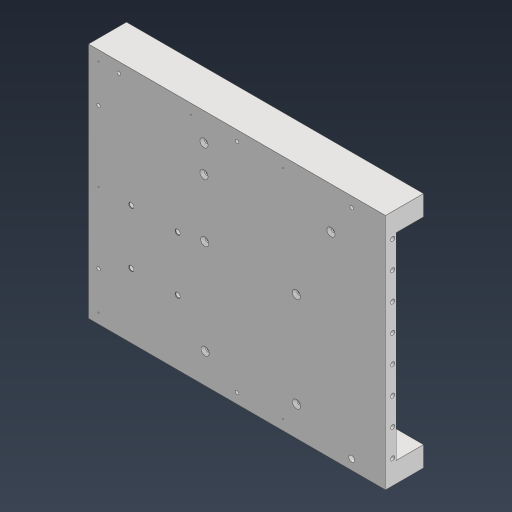
# Autodesk Inventor part: case1
Saved by Autodesk Inventor 2023 (Build 270158000, 158)
## iProperties
Created: 2026-01-23
Part Number: case1
Material: Generic
Document SubType Name: Modeling
Designer: szymo
Density: 1 g/cm^3
Appearance: Default
Author: szymo
Autodesk Inventor part; units mm, degrees
sketch "Sketch1" plane through (0, 0, 0) normal (0, 0, 1) x (1, 0, 0)
  line L0 (100, -105) -> (100, 95)
  line L1 (100, 95) -> (-150, 95)
  line L2 (-150, 95) -> (-150, -105)
  line L3 (-150, -105) -> (100, -105)
  line L4 (-150, -105) -> (-400, -105)
  line L5 (-400, -105) -> (-400, 95)
  line L6 (-400, 95) -> (-150, 95)
  line L7 (-150, 95) -> (-150, -105)
  line L8 (-150, -88) -> (-400, -88)
  line L9 (-400, 78) -> (-150, 78)
  line L10 (-150, -88) -> (83, -88)
  line L11 (83, 78) -> (-150, 78)
  line L12 (-150, 78) -> (-150, 78)
  line L13 (-150, -88) -> (-150, -88)
  line L14 (-383, -105) -> (-383, 95)
  circle A0 centre (13.833333, -96.5) radius 0.5
  circle A1 centre (91.5, 86.5) radius 0.5
  circle A2 centre (91.5, -96.5) radius 0.5
  circle A3 centre (-63.833333, -96.5) radius 0.5
  circle A4 centre (91.5, -5) radius 0.5
  circle A5 centre (13.833333, 86.5) radius 0.5
  circle A6 centre (-63.833333, 86.5) radius 0.5
  circle A7 centre (-121.5, 86.5) radius 1.5
  circle A8 centre (-25, -96.5) radius 1.5
  circle A9 centre (91.5, 40.75) radius 1.5
  circle A10 centre (74.5, -96.5) radius 1.5
  circle A11 centre (91.5, -50.75) radius 1.5
  circle A12 centre (74.5, 86.5) radius 1.5
  circle A13 centre (-121.5, -96.5) radius 1.5
  circle A14 centre (-25, 86.5) radius 1.5
  point P0 (0, 0)
  point P1 (-125, 125)
  point P2 (-127, 93)
  point P3 (-127, 93)
  point P4 (105, -105)
  point P5 (-383, -88)
  point P6 (-383, 78)
  dimension "d0" = 250
  dimension "d23" = 17
  dimension "d24" = 17
  constraints: 18 end point, 6 point on line, 4 perpendicular, 3 horizontal, 2 parallel
  measures "d0" distance of L1.end L5.end
  measures "d23" distance between parallel lines of L11 L1
  measures "d24" distance between parallel lines of L5 L14
ref_plane "Work Plane1" through (-125, -125, -32) normal (0, 0, -1) x (0, 1, 0)
ref_plane "Work Plane5" through (-127, -103, -32) normal (0, 0, -1) x (0, 1, 0)
extrude "Extrusion1" add sketch "Sketch1" against normal up to surface (32 mm away) contours L4 L14 L8 L2 | L2 L9 L14 L6 | L4 L5 L8 L14 | L14 L9 L5 L6 | L8 L5 L9 L14
ref_plane "Work Plane3" through (-122.5, -105, -3) normal (0, 0, -1) x (0, 1, 0)
sketch "Sketch2" plane through (0, 0, 0) normal (0, 0, 1) x (1, 0, 0)
  line L0 (100, 95) -> (100, -105)
  line L1 (100, -105) -> (-150, -105)
  line L2 (-150, -105) -> (-150, -88)
  line L3 (-150, -88) -> (83, -88)
  line L4 (83, -88) -> (83, 78)
  line L5 (83, 78) -> (-150, 78)
  line L6 (-150, 78) -> (-150, 95)
  line L7 (-150, 95) -> (100, 95)
  line L8 (-150, -105) -> (-400, -105)
  line L9 (-400, -105) -> (-400, 95)
  line L10 (-400, 95) -> (-150, 95)
  line L11 (-150, 95) -> (-150, -105)
  circle A0 centre (13.833333, -96.5) radius 0.5
  circle A1 centre (91.5, 86.5) radius 0.5
  circle A2 centre (91.5, -96.5) radius 0.5
  circle A3 centre (-63.833333, -96.5) radius 0.5
  circle A4 centre (91.5, -5) radius 0.5
  circle A5 centre (13.833333, 86.5) radius 0.5
  circle A6 centre (-63.833333, 86.5) radius 0.5
  circle A7 centre (-121.5, 86.5) radius 1.5
  circle A8 centre (-25, -96.5) radius 1.5
  circle A9 centre (91.5, 40.75) radius 1.5
  circle A10 centre (74.5, -96.5) radius 1.5
  circle A11 centre (91.5, -50.75) radius 1.5
  circle A12 centre (74.5, 86.5) radius 1.5
  circle A13 centre (-121.5, -96.5) radius 1.5
  circle A14 centre (-25, 86.5) radius 1.5
  point P0 (0, 0)
  dimension "d15" = 250
  constraints: 8 end point, 2 parallel, 1 horizontal, 1 perpendicular
  measures "d15" distance between parallel lines of L11 L9
extrude "Extrusion2" add sketch "Sketch2" against normal up to surface (3 mm away) contours L6 L11 L2 L8 L9 L10
sketch "Sketch6" plane through (-150, 78, -3) normal (0, 0, -1) x (-1, 0, 0)
  line L0 (0, 0) -> (233, 0) projected
  line L1 (0, -166) -> (0, 0) projected
  line L2 (233, -166) -> (0, -166) projected
  line L3 (0, -166) -> (233, -166) projected
  line L4 (0, -166) -> (2.5, -166)
  line L5 (2.5, -166) -> (2.5, 0)
  line L6 (2.5, 0) -> (0, 0)
  line L7 (0, 0) -> (0, -166)
  line L8 (36, -166) -> (66, -166)
  line L9 (66, 0) -> (36, 0)
  line L10 (17.5, -166) -> (32.5, -166)
  line L11 (32.5, -166) -> (32.5, 0)
  line L12 (32.5, 0) -> (17.5, 0)
  line L13 (17.5, 0) -> (17.5, -166)
  line L14 (233, 0) -> (233, -166) projected
  point P0 (-150, -78)
  point P1 (250, -164)
  point P2 (17.5, 0)
  point P3 (17.5, -166)
  point P4 (32.5, -166)
  point P5 (32.5, 0)
  dimension "d16" = 2.5
  dimension "d21" = 15
  dimension "d22" = 15
  constraints: 20 end point, 5 parallel, 3 horizontal, 3 point on line, 2 perpendicular, 3 other
  measures "d16" distance between parallel lines of L1 L5
  measures "d21" distance between parallel lines of L13 L5
  measures "d22" distance between parallel lines of L11 L13
ref_plane "Work Plane6" through (-94.5, -85, -9) normal (0, 0, -1) x (0, 1, 0)
extrude "Extrusion6" add sketch "Sketch6" along normal up to surface (6 mm away) contours L0 L5 L2 L1 | L0 L11 L2 L13
sketch "Sketch7" plane through (-400, -105, 0) normal (-1, 0, 0) x (0, 0, 1)
  line L0 (-32, 17) -> (-32, 183)
  line L1 (0, 0) -> (0, 200)
  line L2 (-32, 91.5) -> (0, 91.5)
  line L3 (0, 91.5) -> (0, 108.5)
  line L4 (0, 108.5) -> (-32, 108.5)
  line L5 (-32, 108.5) -> (-32, 91.5)
  line L6 (0, 0) -> (-32, 0)
  line L7 (0, 200) -> (-32, 200)
  line L8 (-22.75, 87.025535) -> (-15, 91.5)
  line L9 (-15, 91.5) -> (-7.25, 87.025535)
  line L10 (-7.25, 87.025535) -> (-7.25, 78.076606)
  line L11 (-7.25, 78.076606) -> (-15, 73.602142)
  line L12 (-15, 73.602142) -> (-22.75, 78.076606)
  line L13 (-22.75, 78.076606) -> (-22.75, 87.025535)
  line L14 (-22.75, 66.127677) -> (-15, 70.602142)
  line L15 (-15, 70.602142) -> (-7.25, 66.127677)
  line L16 (-7.25, 66.127677) -> (-7.25, 57.178748)
  line L17 (-7.25, 57.178748) -> (-15, 52.704283)
  line L18 (-15, 52.704283) -> (-22.75, 57.178748)
  line L19 (-22.75, 57.178748) -> (-22.75, 66.127677)
  line L20 (-22.75, 121.923394) -> (-15, 126.397858)
  line L21 (-15, 126.397858) -> (-7.25, 121.923394)
  line L22 (-7.25, 121.923394) -> (-7.25, 112.974465)
  line L23 (-7.25, 112.974465) -> (-15, 108.5)
  line L24 (-15, 108.5) -> (-22.75, 112.974465)
  line L25 (-22.75, 112.974465) -> (-22.75, 121.923394)
  line L26 (-22.75, 142.821252) -> (-15, 147.295717)
  line L27 (-15, 147.295717) -> (-7.25, 142.821252)
  line L28 (-7.25, 142.821252) -> (-7.25, 133.872323)
  line L29 (-7.25, 133.872323) -> (-15, 129.397858)
  line L30 (-15, 129.397858) -> (-22.75, 133.872323)
  line L31 (-22.75, 133.872323) -> (-22.75, 142.821252)
  line L32 (-3, 43.661423) -> (-3, 184.946283) construction
  point P0 (0, 105)
  point P1 (-15, 82.551071)
  point P2 (-15, 61.653212)
  point P3 (-15, 117.448929)
  point P4 (-15, 138.346788)
  dimension "d25" = 17
  dimension "d26" = 91.5
  dimension "d27" = 91.5
  dimension "d28" = 15.5
  dimension "d29" = 15.5
  dimension "d30" = 15.5
  dimension "d31" = 15.5
  dimension "d34" = 3
  dimension "d35" = 12
  dimension "d36" = 12
  dimension "d37" = 17
  dimension "d38" = 12
  dimension "d39" = 3
  dimension "d40" = 3
  constraints: 58 end point, 5 point on line, 5 vertical, 2 parallel, 1 horizontal, 1 perpendicular, 52 other
  measures "d25" distance of L3.end L2.end
  measures "d26" distance between parallel lines of L6 L2
  measures "d27" distance between parallel lines of L7 L4
  measures "d28" distance between parallel lines of L16 L19
  measures "d29" distance between parallel lines of L13 L10
  measures "d30" distance between parallel lines of L25 L22
  measures "d31" distance between parallel lines of L31 L28
  measures "d34" distance between parallel lines of L32 L1
  measures "d35" distance from line of L32 point (-15, 61.653)
  measures "d36" distance from line of L32 point (-15, 82.551)
  measures "d37" distance from line of L0 point (-15, 61.653)
  measures "d38" distance from line of L32 point (-15, 117.449)
  measures "d39" distance of L20.end L29.end
  measures "d40" distance of L14.end L11.end
extrude "Extrusion7" cut sketch "Sketch7" against normal blind 13.5 contours L24 L25 L20 L21 L22 L23 | L9 L10 L11 L12 L13 L8 | L14 L15 L16 L17 L18 L19 | L26 L27 L28 L29 L30 L31
sketch "Sketch8" plane through (-386.5, -105, 0) normal (-1, 0, 0) x (0, 0, 1)
  line L0 (-15, 52.704283) -> (-22.75, 57.178748) construction
  line L1 (-7.25, 57.178748) -> (-15, 52.704283) construction
  line L2 (-7.25, 66.127677) -> (-7.25, 57.178748) construction
  line L3 (-15, 70.602142) -> (-7.25, 66.127677) construction
  line L4 (-22.75, 66.127677) -> (-15, 70.602142) construction
  line L5 (-22.75, 57.178748) -> (-22.75, 66.127677) construction
  line L6 (-15, 73.602142) -> (-22.75, 78.076606) construction
  line L7 (-7.25, 78.076606) -> (-15, 73.602142) construction
  line L8 (-7.25, 87.025535) -> (-7.25, 78.076606) construction
  line L9 (-15, 91.5) -> (-7.25, 87.025535) construction
  line L10 (-22.75, 87.025535) -> (-15, 91.5) construction
  line L11 (-22.75, 78.076606) -> (-22.75, 87.025535) construction
  line L12 (-15, 126.397858) -> (-7.25, 121.923394) construction
  line L13 (-22.75, 121.923394) -> (-15, 126.397858) construction
  line L14 (-22.75, 112.974465) -> (-22.75, 121.923394) construction
  line L15 (-15, 108.5) -> (-22.75, 112.974465) construction
  line L16 (-7.25, 112.974465) -> (-15, 108.5) construction
  line L17 (-7.25, 121.923394) -> (-7.25, 112.974465) construction
  line L18 (-15, 129.397858) -> (-22.75, 133.872323) construction
  line L19 (-7.25, 133.872323) -> (-15, 129.397858) construction
  line L20 (-7.25, 142.821252) -> (-7.25, 133.872323) construction
  line L21 (-15, 147.295717) -> (-7.25, 142.821252) construction
  line L22 (-22.75, 142.821252) -> (-15, 147.295717) construction
  line L23 (-22.75, 133.872323) -> (-22.75, 142.821252) construction
  line L24 (-22.75, 57.178748) -> (-7.25, 66.127677) construction
  line L25 (-7.25, 57.178748) -> (-22.75, 66.127677) construction
  line L26 (-22.75, 78.076606) -> (-7.25, 87.025535) construction
  line L27 (-7.25, 78.076606) -> (-22.75, 87.025535) construction
  line L28 (-22.75, 112.974465) -> (-7.25, 121.923394) construction
  line L29 (-22.75, 121.923394) -> (-15, 126.397858) construction
  line L30 (-7.25, 112.974465) -> (-22.75, 121.923394) construction
  line L31 (-22.75, 133.872323) -> (-7.25, 142.821252) construction
  line L32 (-7.25, 133.872323) -> (-22.75, 142.821252) construction
  circle A0 centre (-15, 61.653212) radius 6
  circle A1 centre (-15, 82.551071) radius 6
  circle A2 centre (-15, 117.448929) radius 6
  circle A3 centre (-15, 138.346788) radius 6
  point P0 (0, 105)
  dimension "d43" = 12
  dimension "d44" = 12
  dimension "d45" = 12
  dimension "d46" = 12
  constraints: 16 end point, 4 centre point, 4 midpoint, 4 parallel, 1 point on line
  measures "d43" diameter of A0
  measures "d44" diameter of A1
  measures "d45" diameter of A2
  measures "d46" diameter of A3
extrude "Extrusion8" cut sketch "Sketch8" against normal blind 13.5
chamfer "Chamfer1" distance 1 angle 45 28 edges at (-400, -43.3468, -22.75) (-400, -36.6351, -18.875) (-400, -36.6351, -11.125) (-400, -43.3468, -7.25) (-400, -50.0585, -11.125) (-400, -50.0585, -18.875) (-386.5, -43.3468, -21) (-386.5, -22.4489, -21) (-400, -29.1606, -18.875) (-400, -29.1606, -11.125) (-400, -22.4489, -7.25) (-400, -15.7372, -11.125) (-400, -15.7372, -18.875) (-400, -22.4489, -22.75) (-400, 12.4489, -22.75) (-400, 5.7372, -18.875) (-400, 5.7372, -11.125) (-400, 19.1606, -11.125) (-400, 12.4489, -7.25) (-400, 19.1606, -18.875) (-400, 26.6351, -18.875) (-400, 26.6351, -11.125) (-400, 33.3468, -7.25) (-400, 40.0585, -11.125) (-400, 40.0585, -18.875) (-400, 33.3468, -22.75) (-386.5, 33.3468, -21) (-386.5, 12.4489, -21)
sketch "Sketch9" plane through (-400, -105, 0) normal (0, -1, 0) x (1, 0, 0)
  line L0 (87.714272, -1.774047) -> (92.175, -6)
  arc A0 (87.714272, -1.774047) -> (87.026528, -1.5) centre (87.026528, -2.5) ccw
  line L1 (63.823472, -1.5) -> (87.026528, -1.5)
  arc A1 (63.823472, -1.5) -> (63.135728, -1.774047) centre (63.823472, -2.5) ccw
  line L2 (63.135728, -1.774047) -> (58.675, -6)
  line L3 (58.675, -6) -> (56.175, -6)
  arc A2 (56.175, -6) -> (54.175, -8) centre (56.175, -8) ccw
  line L4 (54.175, -8) -> (54.175, -14)
  arc A3 (54.175, -14) -> (56.175, -16) centre (56.175, -14) ccw
  line L5 (56.175, -16) -> (58.675, -16)
  line L6 (58.675, -16) -> (63.135728, -20.225953)
  arc A4 (63.135728, -20.225953) -> (63.823472, -20.5) centre (63.823472, -19.5) ccw
  line L7 (87.026528, -20.5) -> (63.823472, -20.5)
  arc A5 (87.026528, -20.5) -> (87.714272, -20.225953) centre (87.026528, -19.5) ccw
  line L8 (92.175, -16) -> (87.714272, -20.225953)
  line L9 (94.675, -16) -> (92.175, -16)
  arc A6 (94.675, -16) -> (96.675, -14) centre (94.675, -14) ccw
  line L10 (96.675, -8) -> (96.675, -14)
  arc A7 (96.675, -8) -> (94.675, -6) centre (94.675, -8) ccw
  line L11 (92.175, -6) -> (94.675, -6)
  circle A8 centre (91.775, -11) radius 3.5
  circle A9 centre (59.075, -11) radius 3.5
  line L12 (65.275, -16.5) -> (83.575, -16.5)
  arc A10 (64.275, -15.5) -> (65.275, -16.5) centre (65.275, -15.5) ccw
  line L13 (64.275, -15.5) -> (64.275, -6.5)
  arc A11 (65.275, -5.5) -> (64.275, -6.5) centre (65.275, -6.5) ccw
  line L14 (83.575, -5.5) -> (65.275, -5.5)
  line L15 (86.575, -8.5) -> (83.575, -5.5)
  line L16 (86.575, -13.5) -> (86.575, -8.5)
  line L17 (83.575, -16.5) -> (86.575, -13.5)
  arc A12 (62.791856, -20.588929) -> (63.823472, -21) centre (63.823472, -19.5) ccw
  line L18 (62.791856, -20.588929) -> (58.475764, -16.5)
  line L19 (58.475764, -16.5) -> (56.175, -16.5)
  arc A13 (53.675, -14) -> (56.175, -16.5) centre (56.175, -14) ccw
  line L20 (53.675, -14) -> (53.675, -8)
  arc A14 (56.175, -5.5) -> (53.675, -8) centre (56.175, -8) ccw
  line L21 (56.175, -5.5) -> (58.475764, -5.5)
  line L22 (58.475764, -5.5) -> (62.791856, -1.411071)
  arc A15 (63.823472, -1) -> (62.791856, -1.411071) centre (63.823472, -2.5) ccw
  line L23 (63.823472, -1) -> (87.026528, -1)
  arc A16 (88.058144, -1.411071) -> (87.026528, -1) centre (87.026528, -2.5) ccw
  line L24 (88.058144, -1.411071) -> (92.374236, -5.5)
  line L25 (92.374236, -5.5) -> (94.675, -5.5)
  arc A17 (97.175, -8) -> (94.675, -5.5) centre (94.675, -8) ccw
  line L26 (97.175, -8) -> (97.175, -14)
  arc A18 (94.675, -16.5) -> (97.175, -14) centre (94.675, -14) ccw
  line L27 (94.675, -16.5) -> (92.374236, -16.5)
  line L28 (92.374236, -16.5) -> (88.058144, -20.588929)
  arc A19 (87.026528, -21) -> (88.058144, -20.588929) centre (87.026528, -19.5) ccw
  line L29 (87.026528, -21) -> (63.823472, -21)
  point P0 (400, 0)
  dimension "d52" = 0.5
  constraints: 24 end point, 16 point on circle, 8 centre point, 19 other
  measures "d52" distance between parallel lines of L7 L29
extrude "Extrusion9" cut sketch "Sketch9" against normal blind 7 contours L0 L11 A7 L10 A6 L9 L8 A5 L7 A4 L6 L5 A3 L4 A2 L3 L2 A1 L1 A0 | A8 | A9 | A10 L13 A11 L14 L15 L16 L17 L12 | L18 L19 A13 L20 A14 L21 L22 A15 L23 A16 L24 L25 A17 L26 A18 L27 L28 A19 L29 A12
sketch "Sketch10" plane through (-400, -98, 0) normal (0, -1, 0) x (1, 0, 0)
  line L0 (64.425, -4) -> (84.425, -4) projected
  line L1 (84.425, -4) -> (87.925, -7.5) projected
  line L2 (87.925, -7.5) -> (87.925, -14.5) projected
  line L3 (87.925, -14.5) -> (84.425, -18) projected
  line L4 (84.425, -18) -> (64.425, -18) projected
  arc A0 (62.925, -16.5) -> (64.425, -18) centre (64.425, -16.5) ccw projected
  line L5 (62.925, -16.5) -> (62.925, -5.5) projected
  arc A1 (64.425, -4) -> (62.925, -5.5) centre (64.425, -5.5) ccw projected
  circle A2 centre (70.125, -11) radius 4.5 projected
  circle A3 centre (80.725, -11) radius 4.5 projected
  point P0 (400, 0)
extrude "Extrusion10" cut sketch "Sketch10" against normal blind 75.75 contours L0 L1 L2 L3 L4 A0 L5 A1 | A2 | A3
chamfer "Chamfer2" distance 1 angle 45 8 edges at (-325.575, -98, -18) (-336.6357, -98, -17.5607) (-337.075, -98, -11) (-336.6357, -98, -4.4393) (-325.575, -98, -4) (-313.825, -98, -16.25) (-312.075, -98, -11) (-313.825, -98, -5.75)
sketch "Sketch11" plane through (-400, -105, 0) normal (0, -1, 0) x (1, 0, 0)
  line L0 (87.026528, -21) -> (63.823472, -21)
  arc A0 (62.791856, -20.588929) -> (63.823472, -21) centre (63.823472, -19.5) ccw
  line L1 (62.791856, -20.588929) -> (58.475764, -16.5)
  line L2 (58.475764, -16.5) -> (56.175, -16.5)
  arc A1 (53.675, -14) -> (56.175, -16.5) centre (56.175, -14) ccw
  line L3 (53.675, -14) -> (53.675, -8)
  arc A2 (56.175, -5.5) -> (53.675, -8) centre (56.175, -8) ccw
  line L4 (56.175, -5.5) -> (58.475764, -5.5)
  line L5 (58.475764, -5.5) -> (62.791856, -1.411071)
  arc A3 (63.823472, -1) -> (62.791856, -1.411071) centre (63.823472, -2.5) ccw
  line L6 (63.823472, -1) -> (87.026528, -1)
  arc A4 (88.058144, -1.411071) -> (87.026528, -1) centre (87.026528, -2.5) ccw
  line L7 (88.058144, -1.411071) -> (92.374236, -5.5)
  line L8 (92.374236, -5.5) -> (94.675, -5.5)
  arc A5 (97.175, -8) -> (94.675, -5.5) centre (94.675, -8) ccw
  line L9 (97.175, -8) -> (97.175, -14)
  arc A6 (94.675, -16.5) -> (97.175, -14) centre (94.675, -14) ccw
  line L10 (94.675, -16.5) -> (92.374236, -16.5)
  line L11 (92.374236, -16.5) -> (88.058144, -20.588929)
  arc A7 (87.026528, -21) -> (88.058144, -20.588929) centre (87.026528, -19.5) ccw
  line L12 (0, 0) -> (0, -32)
  line L13 (0, -32) -> (250, -32)
  line L14 (250, 0) -> (250, -32)
  line L15 (0, 0) -> (250, 0)
  line L16 (110.675, -1) -> (40.175, -1)
  line L17 (40.175, -1) -> (40.175, -26)
  line L18 (40.175, -26) -> (110.675, -26)
  line L19 (110.675, -26) -> (110.675, -1)
  point P0 (400, 0)
  point P1 (63.823472, -1)
  point P2 (58.823472, -21)
  point P3 (87.026528, -1)
  dimension "d60" = 0
  dimension "d61" = 13.5
  dimension "d62" = 13.5
  dimension "d68" = 5
  constraints: 8 end point, 2 parallel, 1 horizontal, 1 perpendicular
  measures "d60" distance between parallel lines of L16 L6
  measures "d61" distance between parallel lines of L19 L9
  measures "d62" distance between parallel lines of L17 L3
  measures "d68" distance between parallel lines of L18 L0
extrude "Extrusion11" cut sketch "Sketch11" against normal blind 3 contours A7 L11 L10 A6 L9 A5 L8 L7 A4 L16 L19 L18 L17 A3 L5 L4 A2 L3 A1 L2 L1 A0 L0
sketch "Sketch12" plane through (-150, -105, -32) normal (0, 0, -1) x (-1, 0, 0)
  line L0 (139.325, 3) -> (209.825, 3)
  line L1 (0, 17) -> (233, 17)
  line L2 (139.325, 3.4) -> (209.825, 3.4) construction
  line L3 (162.973472, 3) -> (139.325, 3)
  line L4 (139.325, 3) -> (139.325, 3.4) construction
  line L5 (209.825, 3) -> (209.825, 3.4) construction
  line L6 (152.825, 3) -> (155.325, 3)
  line L7 (152.825, 3) -> (152.825, 7.391721) construction
  line L8 (196.325, 3) -> (196.325, 7) construction
  line L9 (196.325, 3) -> (196.325, 7)
  line L10 (141.325, 3.4) -> (150.825, 3.4)
  line L11 (150.825, 3.4) -> (150.825, 8.8)
  line L12 (150.825, 8.8) -> (141.325, 8.8)
  line L13 (141.325, 8.8) -> (141.325, 3.4)
  line L14 (207.825, 3.4) -> (198.325, 3.4)
  line L15 (198.325, 3.4) -> (198.325, 8.8)
  line L16 (198.325, 8.8) -> (207.825, 8.8)
  line L17 (207.825, 8.8) -> (207.825, 3.4)
  point P0 (-150, 105)
  dimension "d69" = 0.4
  dimension "d70" = 2
  dimension "d71" = 2
  dimension "d72" = 9.5
  dimension "d73" = 5.4
  dimension "d76" = 9.5
  dimension "d77" = 2
  dimension "d78" = 5.4
  constraints: 26 end point, 4 parallel, 3 horizontal, 3 perpendicular, 3 vertical, 2 point on line
  measures "d69" distance between parallel lines of L2 L0
  measures "d70" distance between parallel lines of L4 L13
  measures "d71" distance between parallel lines of L11 L7
  measures "d72" distance of L11.end L12.end
  measures "d73" distance between parallel lines of L12 L10
  measures "d76" distance of L15.end L16.end
  measures "d77" distance between parallel lines of L8 L15
  measures "d78" distance between parallel lines of L2 L16
extrude "Extrusion12" cut sketch "Sketch12" against normal blind 27
chamfer "Chamfer4" distance 1 angle 45 8 edges at (-296.075, -96.2, -32) (-291.325, -98.9, -32) (-296.075, -101.6, -32) (-300.825, -98.9, -32) (-353.075, -96.2, -32) (-348.325, -98.9, -32) (-353.075, -101.6, -32) (-357.825, -98.9, -32)
sketch "Sketch13" plane through (-400, -105, 0) normal (0, -1, 0) x (1, 0, 0)
  line L0 (0, 0) -> (0, -32) projected
  line L1 (0, -32) -> (250, -32) projected
  line L2 (250, 0) -> (250, -32) projected
  line L3 (0, 0) -> (250, 0) projected
  line L4 (40.175, -1) -> (110.675, -1) projected
  line L5 (110.675, -1) -> (110.675, -26) projected
  line L6 (110.675, -26) -> (40.175, -26) projected
  line L7 (40.175, -26) -> (40.175, -1) projected
  circle A0 centre (27.175, -15) radius 10
  point P0 (400, 0)
  dimension "d82" = 20
  dimension "d83" = 5
  dimension "d84" = 3
  dimension "d85" = 17.175
  dimension "d91" = 15
  constraints: 1 centre point
  measures "d82" diameter of A0
  measures "d83" distance edge to line of A0 L3
  measures "d84" distance edge to line of A0 L7
  measures "d85" distance edge to line of A0 L0
  measures "d91" distance from line of L3 A0.centre
extrude "Extrusion13" cut sketch "Sketch13" against normal blind 5 contours A0
sketch "Sketch14" plane through (-372.825, -100, -15) normal (0, -1, 0) x (1, 0, 0)
  circle A0 centre (0, 0) radius 10 projected
  circle A1 centre (0, 0) radius 7.5
  point P0 (372.825, 15)
  dimension "d88" = 15
  constraints: 1 centre point, 1 coincident
  measures "d88" diameter of A1
extrude "Extrusion14" cut sketch "Sketch14" against normal blind 16 contours A1
chamfer "Chamfer5" distance 1 angle 45 1 edges at (-380.325, -100, -15)
chamfer "Chamfer6" distance 1 angle 45 19 edges at (-324.575, -102, -21) (-312.4182, -102, -20.8934) (-309.7838, -102, -18.5445) (-336.7318, -102, -20.8934) (-339.3662, -102, -18.5445) (-342.6746, -102, -16.5) (-345.5928, -102, -15.7678) (-346.325, -102, -11) (-345.5928, -102, -6.2322) (-342.6746, -102, -5.5) (-339.3662, -102, -3.4555) (-336.7318, -102, -1.1066) (-309.7838, -102, -3.4555) (-312.4182, -102, -1.1066) (-306.4754, -102, -5.5) (-303.5572, -102, -6.2322) (-302.825, -102, -11) (-303.5572, -102, -15.7678) (-306.4754, -102, -16.5)
sketch "Sketch15" plane through (-383, -88, -32) normal (0, 1, 0) x (1, 0, 0)
  line L0 (70.714272, -30.225953) -> (75.175, -26)
  arc A0 (70.026528, -30.5) -> (70.714272, -30.225953) centre (70.026528, -29.5) ccw
  line L1 (46.823472, -30.5) -> (70.026528, -30.5)
  arc A1 (46.135728, -30.225953) -> (46.823472, -30.5) centre (46.823472, -29.5) ccw
  line L2 (46.135728, -30.225953) -> (41.675, -26)
  line L3 (41.675, -26) -> (39.175, -26)
  arc A2 (37.175, -24) -> (39.175, -26) centre (39.175, -24) ccw
  line L4 (37.175, -24) -> (37.175, -18)
  arc A3 (39.175, -16) -> (37.175, -18) centre (39.175, -18) ccw
  line L5 (39.175, -16) -> (41.675, -16)
  line L6 (41.675, -16) -> (46.135728, -11.774047)
  arc A4 (46.823472, -11.5) -> (46.135728, -11.774047) centre (46.823472, -12.5) ccw
  line L7 (70.026528, -11.5) -> (46.823472, -11.5)
  arc A5 (70.714272, -11.774047) -> (70.026528, -11.5) centre (70.026528, -12.5) ccw
  line L8 (75.175, -16) -> (70.714272, -11.774047)
  line L9 (77.675, -16) -> (75.175, -16)
  arc A6 (79.675, -18) -> (77.675, -16) centre (77.675, -18) ccw
  line L10 (79.675, -24) -> (79.675, -18)
  arc A7 (77.675, -26) -> (79.675, -24) centre (77.675, -24) ccw
  line L11 (75.175, -26) -> (77.675, -26)
  circle A8 centre (74.775, -21) radius 3.5
  circle A9 centre (42.075, -21) radius 3.5
  line L12 (48.275, -15.5) -> (66.575, -15.5)
  arc A10 (48.275, -15.5) -> (47.275, -16.5) centre (48.275, -16.5) ccw
  line L13 (47.275, -16.5) -> (47.275, -25.5)
  arc A11 (47.275, -25.5) -> (48.275, -26.5) centre (48.275, -25.5) ccw
  line L14 (66.575, -26.5) -> (48.275, -26.5)
  line L15 (69.575, -23.5) -> (66.575, -26.5)
  line L16 (69.575, -18.5) -> (69.575, -23.5)
  line L17 (66.575, -15.5) -> (69.575, -18.5)
  point P0 (383, -32)
  constraints: 2 coincident
hole "Hole1" at (-340.925, -88, -11) at (-308.225, -88, -11) direction (0, -1, 0) diameter 4 end through all counterbore diameter 4.5 counterbore depth 1
sketch "Sketch16" plane through (-152.5, -88, -3) normal (-1, 0, 0) x (0, 0, 1)
  line L0 (-6, 166) -> (-6, 0)
  line L1 (0, 0) -> (-6, 0)
  line L2 (0, 166) -> (0, 0)
  line L3 (-6, 166) -> (0, 166)
  circle A0 centre (-3, 3) radius 3
  circle A1 centre (-3, 25.857143) radius 3
  circle A2 centre (-3, 71.571429) radius 3
  circle A3 centre (-3, 94.428571) radius 3
  circle A4 centre (-3, 117.285714) radius 3
  circle A5 centre (-3, 140.142857) radius 3
  circle A6 centre (-3, 48.714286) radius 3
  circle A7 centre (-3, 163) radius 3
  point P0 (3, 88)
  dimension "d105" = 6
  dimension "d107" = 6
  dimension "d108" = 6
  dimension "d109" = 6
  dimension "d110" = 6
  dimension "d111" = 6
  dimension "d112" = 6
  dimension "d114" = 22.85714
  dimension "d115" = 22.85714
  dimension "d116" = 22.85714
  dimension "d117" = 22.85714
  dimension "d118" = 22.85714
  dimension "d119" = 22.85714
  dimension "d120" = 22.85714
  constraints: 11 tangent, 8 centre point, 8 coincident
  measures "d105" diameter of A0
  measures "d107" diameter of A1
  measures "d108" diameter of A2
  measures "d109" diameter of A3
  measures "d110" diameter of A4
  measures "d111" diameter of A5
  measures "d112" diameter of A6
  measures "d114" distance of A1.centre A0.centre
  measures "d115" distance of A6.centre A1.centre
  measures "d116" distance of A2.centre A6.centre
  measures "d117" distance of A3.centre A2.centre
  measures "d118" distance of A4.centre A3.centre
  measures "d119" distance of A5.centre A4.centre
  measures "d120" distance of A7.centre A5.centre
hole "Hole2" at (-152.5, -85, -6) at (-152.5, -62.142857, -6) at (-152.5, -39.285714, -6) at (-152.5, -16.428571, -6) at (-152.5, 6.428571, -6) at (-152.5, 29.285714, -6) at (-152.5, 52.142857, -6) at (-152.5, 75, -6) direction (1, 0, 0) diameter 3.6 end through all clearance for "Countersunk Flat Head Screw ISO 2009/7046" size "M3" standard "ISO"
hole "Hole3" at (-301.809738, -79.8167, 0) at (-224.925, -79.925, 0) at (-225.076125, -0.025, 0) at (-195.9, 60, 0) at (-302.749939, 71.5, 0) at (-302.749939, 48.5, 0) at (-302.187779, -0.025, 0) direction (0, 0, -1) diameter 3 end through all countersink diameter 7 countersink angle 90 clearance for "Countersunk Flat Head Screw ISO 2009/7046" size "M3" standard "ISO"
sketch "Sketch18" plane through (0, 0, 0) normal (0, 0, 1) x (1, 0, 0)
  circle A0 centre (-325, -50.6) radius 1.8 projected
  circle A1 centre (-325, -4.6) radius 1.8 projected
  circle A2 centre (-364, -4.6) radius 1.8 projected
  circle A3 centre (-364, -50.6) radius 1.8 projected
  point P0 (0, 0)
hole "Hole4" at (-364, -50.6, 0) at (-364, -4.6, 0) at (-325, -4.6, 0) at (-325, -50.6, 0) direction (0, 0, -1) diameter 4 depth 5.5 counterbore diameter 4.5 counterbore depth 0.5
sketch "Sketch19" plane through (-150, -105, -32) normal (0, 0, -1) x (-1, 0, 0)
  line L0 (151.825, 9.8) -> (140.325, 9.8)
  line L1 (151.825, 2.4) -> (151.825, 9.8)
  line L2 (140.325, 2.4) -> (151.825, 2.4)
  line L3 (140.325, 9.8) -> (140.325, 2.4)
  line L4 (250, 0) -> (0, 0)
  line L5 (250, 200) -> (250, 0)
  line L6 (0, 200) -> (250, 200)
  line L7 (0, 183) -> (0, 200)
  line L8 (233, 183) -> (0, 183)
  line L9 (233, 17) -> (233, 183)
  line L10 (0, 17) -> (233, 17)
  line L11 (0, 0) -> (0, 17)
  line L12 (197.325, 2.4) -> (208.825, 2.4)
  line L13 (197.325, 9.8) -> (197.325, 2.4)
  line L14 (208.825, 9.8) -> (197.325, 9.8)
  line L15 (208.825, 2.4) -> (208.825, 9.8)
  line L16 (0, 0) -> (0, 200)
  circle A0 centre (-28.5, 8.5) radius 2.5
  circle A1 centre (-86.166667, 8.5) radius 0.5
  circle A2 centre (-125, 8.5) radius 1.5
  circle A3 centre (-163.833333, 8.5) radius 0.5
  circle A4 centre (-224.5, 8.5) radius 1.5
  circle A5 centre (-241.5, 8.5) radius 0.5
  circle A6 centre (-241.5, 54.25) radius 1.5
  circle A7 centre (-241.5, 100) radius 0.5
  circle A8 centre (-241.5, 145.75) radius 1.5
  circle A9 centre (-241.5, 191.5) radius 0.5
  circle A10 centre (-224.5, 191.5) radius 1.5
  circle A11 centre (-163.833333, 191.5) radius 0.5
  circle A12 centre (-125, 191.5) radius 1.5
  circle A13 centre (-86.166667, 191.5) radius 0.5
  circle A14 centre (-28.5, 191.5) radius 1.5
  circle A15 centre (28.5, 8.5) radius 2.5
  circle A16 centre (86.166667, 8.5) radius 0.5
  circle A17 centre (125, 8.5) radius 1.5
  circle A18 centre (241.5, 8.5) radius 0.5
  circle A19 centre (241.5, 40.5) radius 1.5
  circle A20 centre (241.5, 100) radius 0.5
  circle A21 centre (241.5, 159.5) radius 1.5
  circle A22 centre (241.5, 191.5) radius 0.5
  circle A23 centre (224.5, 191.5) radius 1.5
  circle A24 centre (163.833333, 191.5) radius 0.5
  circle A25 centre (125, 191.5) radius 1.5
  circle A26 centre (86.166667, 191.5) radius 0.5
  circle A27 centre (28.5, 191.5) radius 1.5
  line L17 (233, 17) -> (32.5, 17)
  line L18 (233, 17) -> (250, 17)
  line L19 (233, 183) -> (250, 183)
  circle A28 centre (241.5, 40.5) radius 8.5
  circle A29 centre (241.5, 159.5) radius 8.5
  point P0 (-150, 105)
  point P1 (150, 105)
  dimension "d142" = 17
  dimension "d143" = 17
  dimension "d144" = 3
  dimension "d145" = 3
  dimension "d146" = 15
  dimension "d148" = 23.5
  constraints: 15 centre point, 12 symmetric about line, 6 end point, 2 coincident, 2 perpendicular, 2 point on line, 1 collinear, 11 other
  measures "d142" diameter of A28
  measures "d143" diameter of A29
  measures "d144" diameter of A19
  measures "d145" diameter of A21
  measures "d146" distance edge to line of A28 L18
  measures "d148" distance from line of A29.centre L19
extrude "Extrusion15" cut sketch "Sketch19" against normal through all contours A15 | A16 | A17 | A18 | A19 | A20 | A21 | A22 | A23 | A24 | A25 | A26 | A27
equation "\"d24\" = d23"
equation "\"d26\" = d27"
equation "\"d29\" = d28"
equation "\"d30\" = d28"
equation "\"d31\" = d28"
equation "\"d36\" = d35"
equation "\"d38\" = d35"
equation "\"d39\" = d40"
body "Solid1"
